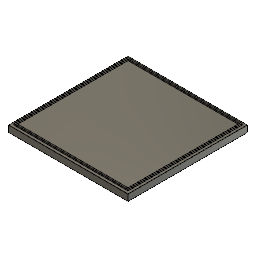
Plate-top (Autodesk Fusion 360 design; units mm, degrees)
Autodesk Fusion 360 part; units mm, degrees
sketch "Sketch1" plane through (0, 0, 0) normal (0, 1, 0) x (1, 0, 0)
  line L0 (-50, 50) -> (130, 50)
  line L1 (130, 50) -> (130, -130)
  line L2 (130, -130) -> (-50, -130)
  line L3 (-50, -130) -> (-50, 50)
  dimension "d1" = 180
  dimension "d2" = 180
  constraint horizontal L0
  constraint vertical L1
  constraint horizontal L2
  constraint vertical L3
  measures "d1" distance of L0.start L0.end
  measures "d2" distance of L0.start L2.end
extrude "Extrude1" add sketch "Sketch1" along normal blind 10
sketch "Sketch2" plane through (0, 10, 0) normal (0, 1, 0) x (-1, 0, 0)
  line L0 (50, 130) -> (-130, 130)
  line L1 (-130, 130) -> (-130, -50)
  line L2 (-130, -50) -> (50, -50)
  line L3 (50, -50) -> (50, 130)
  line L4 (46, 126) -> (-126, 126)
  line L5 (-126, 126) -> (-126, -46)
  line L6 (-126, -46) -> (46, -46)
  line L7 (46, -46) -> (46, 126)
  dimension "d5" = 172
  dimension "d6" = 172
  constraint horizontal L4
  constraint vertical L5
  constraint horizontal L6
  constraint vertical L7
  measures "d5" distance of L4.start L4.end
  measures "d6" distance of L4.start L6.end
extrude "Extrude2" add sketch "Sketch2" along normal blind 2 contours L4 L5 L6 L7
sketch "Sketch3" plane through (0, 12, 0) normal (0, 1, 0) x (-1, 0, 0)
  line L0 (46, -46) -> (46, 126)
  line L1 (46, 126) -> (-126, 126)
  line L2 (-126, 126) -> (-126, -46)
  line L3 (-126, -46) -> (46, -46)
  line L4 (44, 124) -> (-124, 124)
  line L5 (-124, 124) -> (-124, -44)
  line L6 (-124, -44) -> (44, -44)
  line L7 (44, -44) -> (44, 124)
  constraint horizontal L4
  constraint vertical L5
  constraint horizontal L6
  constraint vertical L7
extrude "Extrude3" cut sketch "Sketch3" against normal blind 2 contours L4 L5 L6 L7
